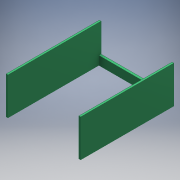
# Autodesk Inventor part: Porte Double
Saved by Autodesk Inventor 2016 SP1 (Build 200210100, 210)
## iProperties
Created: 2016-10-04
Part Number: Porte Double
Material: Bois (Chêne)
Document SubType Name: Modeling
Designer: dimercur
Density: 0.76 g/cm^3
Appearance: Lisse - Vert mer foncé
Mass: 2.41701e+06 g
Surface Area: 140524 cm^2
Volume: 3.18028e+06 cm^3
Author: dimercur
Autodesk Inventor part; units mm, degrees
ref_plane "YZ Plane" through (0, 0, 0) normal (1, 0, 0) x (0, 1, 0)
ref_plane "XZ Plane" through (0, 0, 0) normal (0, 1, 0) x (-1, 0, 0)
ref_plane "XY Plane" through (0, 0, 0) normal (0, 0, 1) x (1, 0, 0)
sketch "Esquisse1" plane through (0, 0, 0) normal (0, 0, 1) x (1, 0, 0)
  line L0 (-954.3902, 760.3659) -> (765.6098, 760.3659)
  line L1 (765.6098, 760.3659) -> (765.6098, -1389.6341)
  line L2 (765.6098, -1389.6341) -> (-954.3902, -1389.6341)
  line L3 (-954.3902, -1389.6341) -> (-954.3902, 760.3659)
  point P0 (0, 0)
  dimension "d0" = 1720
  dimension "d1" = 2150
  constraints: 8 end point, 2 parallel, 1 horizontal, 1 perpendicular
  measures "d0" distance of L0.start L0.end
  measures "d1" distance of L2.end L0.start
extrude "Extrusion1" add sketch "Esquisse1" along normal blind 860
sketch "Esquisse2" plane through (-954.3902, 760.3659, 0) normal (0, 1, 0) x (1, 0, 0)
  line L0 (1720, -860) -> (0, -860) projected
  line L1 (40, -860) -> (1680, -860)
  line L2 (1680, -860) -> (1680, -200)
  line L3 (1680, -200) -> (40, -200)
  line L4 (40, -200) -> (40, -860)
  line L5 (0, 0) -> (1720, 0) projected
  point P0 (954.3902, 0)
  dimension "d4" = 40
  dimension "d5" = 40
  dimension "d6" = 200
  constraints: 8 end point, 2 parallel, 1 horizontal, 1 perpendicular, 1 point on line
  measures "d4" distance of L1.start L0.end
  measures "d5" distance of L0.start L1.end
  measures "d6" distance from line of L5 L3.end
extrude "Extrusion2" cut sketch "Esquisse2" against normal through all
sketch "Esquisse3" plane through (-914.3902, 760.3659, 200) normal (0, 0, 1) x (1, 0, 0)
  line L0 (0, -2150) -> (0, 0) projected
  line L1 (1640, 0) -> (1640, -2150) projected
  line L2 (0, -50) -> (1640, -50)
  line L3 (1640, -50) -> (1640, -2150)
  line L4 (1640, -2150) -> (0, -2150)
  line L5 (0, -2150) -> (0, -50)
  line L6 (0, 0) -> (1640, 0) projected
  point P0 (914.3902, -760.3659)
  dimension "d9" = 50
  constraints: 8 end point, 2 parallel, 1 horizontal, 1 perpendicular, 1 point on line
  measures "d9" distance between parallel lines of L2 L6
extrude "Extrusion3" cut sketch "Esquisse3" against normal blind 1000 contours L0 L2 L1 L4
